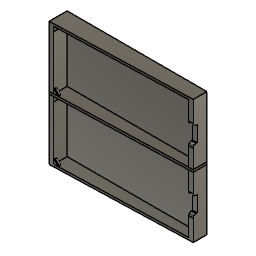
casier_dets_x2 (Autodesk Fusion 360 design; units mm, degrees)
Autodesk Fusion 360 part; units mm, degrees
sketch "Esquisse1" plane through (0, 0, 0) normal (0, 1, 0) x (1, 0, 0)
  line L0 (31, 14) -> (-31, 14)
  line L1 (-31, 14) -> (-31, -14)
  line L2 (-31, -14) -> (31, -14)
  line L3 (31, -14) -> (31, 14)
  line L4 (31, 14) -> (-31, -14) construction
  line L5 (-31, 14) -> (31, -14) construction
  line L6 (29, 13) -> (-29, 13)
  line L7 (-29, 13) -> (-29, -13)
  line L8 (-29, -13) -> (29, -13)
  line L9 (29, -13) -> (29, 13)
  line L10 (29, 13) -> (-29, -13) construction
  line L11 (-29, 13) -> (29, -13) construction
  dimension "d4" = 62
  dimension "d5" = 28
  dimension "d6" = 58
  dimension "d7" = 26
  constraint horizontal L0
  constraint perpendicular L0 L1
  constraint parallel L0 L2
  constraint parallel L1 L3
  constraint coincident L4 origin
  constraint coincident L5 origin
  constraint horizontal L6
  constraint perpendicular L6 L7
  constraint parallel L6 L8
  constraint parallel L7 L9
  constraint coincident L10 origin
  constraint coincident L11 origin
  measures "d4" distance of L1.end L2.end
  measures "d5" distance of L0.end L1.end
  measures "d6" distance of L7.end L8.end
  measures "d7" distance of L6.end L7.end
extrude "Extrusion1" add sketch "Esquisse1" along normal blind 8 contours L0 L1 L2 L3 | L6 L7 L8 L9 makes body 1
sketch "Esquisse2" plane through (0, 0, 0) normal (0, -1, 0) x (1, 0, 0)
  line L0 (31, -14) -> (31, 14)
  line L1 (31, 14) -> (-31, 14)
  line L2 (-31, 14) -> (-31, -14)
  line L3 (-31, -14) -> (31, -14)
  line L4 (29, 13) -> (-29, 13)
  line L5 (-29, 13) -> (-29, -13)
  line L6 (-29, -13) -> (29, -13)
  line L7 (29, -13) -> (29, 13)
  line L8 (29, 13) -> (-29, -13) construction
  line L9 (-29, 13) -> (29, -13) construction
  dimension "d10" = 58
  dimension "d11" = 26
  constraint horizontal L4
  constraint perpendicular L4 L5
  constraint parallel L4 L6
  constraint parallel L5 L7
  constraint coincident L8 origin
  constraint coincident L9 origin
  measures "d10" distance of L5.end L6.end
  measures "d11" distance of L4.end L5.end
extrude "Extrusion2" cut sketch "Esquisse2" against normal blind 6 contours L4 L5 L6 L7 bodies 1
sketch "Esquisse3" plane through (0, 0, 0) normal (0, 1, 0) x (1, 0, 0)
  line L0 (-29, -13) -> (-27, -13)
  line L1 (-27, -13) -> (-29, -11)
  line L2 (-29, 13) -> (-27, 13)
  line L3 (-27, 13) -> (-29, 11)
  line L4 (-29, 11) -> (-29, 13)
  line L5 (-29, -13) -> (-29, -11)
  dimension "d14" = 2
  dimension "d15" = 2
  dimension "d16" = 2
  dimension "d17" = 2
  constraint horizontal L0
  constraint horizontal L2
  constraint perpendicular L0 L5
  measures "d14" distance of L0.start L0.end
  measures "d15" distance of L0.start L1.end
  measures "d16" distance of L2.start L2.end
  measures "d17" distance of L2.start L3.end
extrude "Extrusion3" add sketch "Esquisse3" along normal blind 2 separate body makes body 2 at (-27.6667, 0.6667, 12.3333) makes body 3 at (-27.6667, 0.6667, -12.3333)
fillet "Congé4" radius 1.4 1 edges at (-28, 2, 12) on bodies 2
fillet "Congé5" radius 1.4 1 edges at (-28, 2, -12) on bodies 3
sketch "Esquisse6" plane through (0, 0, -14) normal (0, 0, -1) x (1, 0, 0)
  line L0 (31, 0) -> (-31, 0)
  line L1 (-31, 0) -> (-31, -8)
  line L2 (-31, -8) -> (31, -8)
  line L3 (31, -8) -> (31, 0)
  line L4 (-32, 0) -> (32, -2)
  line L5 (32, -2) -> (32, 2.866)
  line L6 (32, 2.866) -> (-32, 2.866)
  line L7 (-32, 2.866) -> (-32, 0)
  constraint parallel L3 L5
  constraint perpendicular L3 L6
  constraint parallel L3 L7
extrude "Extrusion5" cut sketch "Esquisse6" against normal blind 33 contours L0 L1 L3 L4 | L0 L1 L3 L4 L5 L6 L7 bodies 1 2 3
sketch "Esquisse7" plane through (31, 0, 0) normal (1, 0, 0) x (0, 1, 0)
  line L0 (1.9688, 14) -> (1.9688, -14)
  line L1 (1.9688, -14) -> (8, -14)
  line L2 (8, -14) -> (8, 14)
  line L3 (8, 14) -> (1.9688, 14)
  line L4 (-3.75, 3.5) -> (3.75, 3.5)
  line L5 (3.75, 3.5) -> (3.75, -3.5)
  line L6 (3.75, -3.5) -> (-3.75, -3.5)
  line L7 (-3.75, -3.5) -> (-3.75, 3.5)
  line L8 (-3.75, 3.5) -> (3.75, -3.5) construction
  line L9 (3.75, 3.5) -> (-3.75, -3.5) construction
  dimension "d37" = 7.5
  dimension "d38" = 7
  constraint horizontal L4
  constraint perpendicular L4 L5
  constraint parallel L4 L6
  constraint parallel L5 L7
  constraint coincident L8 origin
  constraint coincident L9 origin
  measures "d37" distance of L5.end L6.end
  measures "d38" distance of L4.end L5.end
extrude "Extrusion6" cut sketch "Esquisse7" against normal blind 2 contours L0 L4 L5 L6 | L0 L4 L6 L7 bodies 1
copy_body "Copier/Coller des corps1" bodies 2 3 1 makes body 4 makes body 5 makes body 6
move_body "Déplacer1" bodies 4 5 6 to x (1, 0, 0) y (0, 1, 0) z (0, 0, 1) at (0, 0, -27)
copy_body "Copier/Coller des corps5" bodies 3 2 1 makes body 7 makes body 8 makes body 9
move_body "Déplacer5" bodies 7 8 9 to x (1, 0, 0) y (0, 1, 0) z (0, 0, 1) at (0, 0, -54)
copy_body "Copier/Coller des corps6" bodies 2 1 3 makes body 10 makes body 11 makes body 12
move_body "Déplacer6" bodies 10 11 12 to x (1, 0, 0) y (0, 1, 0) z (0, 0, 1) at (0, 0, -81)
fillet "Congé7" radius 1.2 8 edges at (30, 1.9375, -3.5) (30, 1.9375, 3.5) (30, 1.9375, -30.5) (30, 1.9375, -23.5) (30, 1.9375, -57.5) (30, 1.9375, -50.5) (30, 1.9375, -84.5) (30, 1.9375, -77.5) on bodies 1 6 9 11
hidden bodies 7 8 9 10 11 12
equation "long_carte = 58 mm"
equation "larg_carte = 26 mm"
equation "ep = 2 mm"
equation "d4 = long_carte + 2 * ep"
equation "d5 = larg_carte + ep"
equation "d6 = long_carte"
equation "d7 = larg_carte"
equation "d8 = 4 * ep"
equation "d10 = long_carte"
equation "d11 = larg_carte"
equation "d12 = -3 * ep"
equation "d14 = ep"
equation "d15 = ep"
equation "d16 = ep"
equation "d17 = ep"
equation "d18 = ep"
equation "d39 = -ep"
